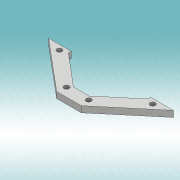
# Autodesk Inventor part: Leg_part1
Saved by Autodesk Inventor 2019 (Build 230136000, 136)
## iProperties
Created: 2019-01-31
Part Number: Leg_part1
Material: Generic
Document SubType Name: Modeling
Designer: nelson.soberon
Density: 1 g/cm^3
Appearance: Default
Author: nelson.soberon
Autodesk Inventor part; units mm, degrees
ref_plane "YZ Plane" through (0, 0, 0) normal (1, 0, 0) x (0, 1, 0)
ref_plane "XZ Plane" through (0, 0, 0) normal (0, 1, 0) x (-1, 0, 0)
ref_plane "XY Plane" through (0, 0, 0) normal (0, 0, 1) x (1, 0, 0)
sketch "Sketch1" plane through (0, 0, 0) normal (0, 0, 1) x (1, 0, 0)
  line L0 (0, 0) -> (-6, 0)
  line L1 (-6, 0) -> (-30.4309, 20.5)
  line L2 (-30.4309, 20.5) -> (-19.4309, 20.5)
  line L3 (-19.4309, 20.5) -> (-19.4309, 19.1023)
  line L4 (-19.4309, 19.1023) -> (-3.8162, 6)
  line L5 (-3.8162, 6) -> (0, 6)
  line L6 (0, 0) -> (0, 6)
  circle A0 centre (-5.4048, 4.2) radius 1.25
  circle A1 centre (-22.7309, 18.1) radius 1.25
  line L7 (0, 0) -> (6, 0)
  line L8 (6, 0) -> (30.4309, 20.5)
  line L9 (30.4309, 20.5) -> (19.4309, 20.5)
  line L10 (19.4309, 20.5) -> (19.4309, 19.1023)
  line L11 (19.4309, 19.1023) -> (3.8162, 6)
  line L12 (3.8162, 6) -> (0, 6)
  circle A2 centre (5.4048, 4.2) radius 1.25
  circle A3 centre (22.7309, 18.1) radius 1.25
  dimension "d6" = 6
  dimension "d8" = 40
  dimension "d9" = 11
  dimension "d10" = 6
  dimension "d12" = 2.5
  dimension "d15" = 2.4
  dimension "d16" = 3.3
  dimension "d17" = 2.4
  dimension "d18" = 4.2
  dimension "d21" = 6
  dimension "d22" = 20.5
  constraints: 28 end point, 7 symmetric about line, 4 centre point, 3 horizontal, 2 perpendicular, 1 equal radius, 1 parallel, 2 other
  measures "d6" distance of L0.start L0.end
  measures "d8" angle of L0 L1
  measures "d9" distance of L1.end L2.end
  measures "d10" distance between parallel lines of L0 L5
  measures "d12" diameter of A0
  measures "d15" distance from line of A1.centre L2
  measures "d16" distance from line of A1.centre L3
  measures "d17" distance from line of L4 A0.centre
  measures "d18" distance from line of L0 A0.centre
  measures "d21" distance between parallel lines of L4 L1
  measures "d22" distance between parallel lines of L0 L2
extrude "Extrusion1" add sketch "Sketch1" along normal mid plane 3
body "Solid1"
